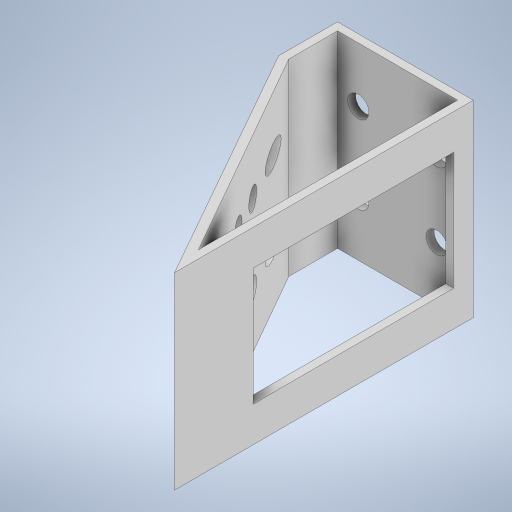
# Autodesk Inventor part: AngleMount
Saved by Autodesk Inventor 2024.2 (Build 282272000, 272)
## iProperties
Created: 2023-11-06
Part Number: AngleMount
Material: Generic
Document SubType Name: Modeling
Designer: S227943
Density: 1 g/cm^3
Appearance: Default
Author: S227943
Autodesk Inventor part; units mm, degrees
ref_plane "YZ Plane" through (0, 0, 0) normal (1, 0, 0) x (0, 1, 0)
ref_plane "XZ Plane" through (0, 0, 0) normal (0, 1, 0) x (-1, 0, 0)
ref_plane "XY Plane" through (0, 0, 0) normal (0, 0, 1) x (1, 0, 0)
sketch "Sketch1" plane through (0, 0, 0) normal (0, 1, 0) x (-1, 0, 0)
  line L0 (0, 0) -> (0, -19.05)
  line L1 (0, -19.05) -> (43.942, -19.05)
  line L2 (43.942, -19.05) -> (43.942, 0)
  line L3 (43.942, 0) -> (0, 0)
  line L4 (0, 0) -> (0, 155.3344)
  line L5 (43.942, 0) -> (0, 77.6672)
  dimension "d0" = 19.05
  dimension "d1" = 43.942
  dimension "d2" = 60.5
  constraints: 12 end point, 2 perpendicular, 2 vertical, 1 horizontal, 1 midpoint
  measures "d0" distance of L0.start L0.end
  measures "d1" distance of L0.end L1.end
  measures "d2" angle of L3 L5
extrude "Extrusion1" add sketch "Sketch1" along normal blind 60.96
sketch "Sketch6" plane through (0, 60.96, 0) normal (0, 1, 0) x (1, 0, 0)
  line L0 (0, 19.05) -> (-43.942, 19.05) projected
  line L1 (0, -76.952) -> (0, 19.05)
  line L2 (0, 19.05) -> (-43.942, 19.05)
  line L3 (-43.942, 19.05) -> (-43.942, 0.0548)
  line L4 (-43.942, 0.0548) -> (0, -76.952)
  line L5 (-2.54, -67.3758) -> (-2.54, 16.51)
  line L6 (-2.54, 16.51) -> (-41.402, 16.51)
  line L7 (-41.402, 16.51) -> (-41.402, 0.7285)
  line L8 (-41.402, 0.7285) -> (-2.54, -67.3758)
  point P0 (0, 0)
  dimension "d26" = 2.54
  constraints: 16 end point, 2 perpendicular, 1 collinear, 1 vertical, 3 other
  measures "d26" distance between parallel lines of L4 L8
extrude "Extrusion5" cut sketch "Sketch6" against normal blind 76.2 contours L8 L7 L6 L5
sketch "Sketch2" plane through (0, 0, 77.6672) normal (-0.8703557, 0, 0.4924236) x (0.4924236, 0, 0.8703557)
  line L0 (0, 60.96) -> (-84.1784, 60.96) projected
  line L1 (0, 60.96) -> (-14.1351, 60.96)
  line L2 (-14.1351, 60.96) -> (-14.1351, 0)
  line L3 (0, 0) -> (-84.1784, 0) projected
  line L4 (-14.1351, 60.96) -> (-75.0951, 60.96)
  line L5 (-75.0951, 60.96) -> (-75.0951, 0)
  line L6 (-75.0951, 0) -> (-14.1351, 0)
  line L7 (-14.1351, 60.96) -> (-44.6151, 60.96)
  line L8 (-44.6151, 60.96) -> (-44.6151, 0)
  line L9 (-75.0951, 30.48) -> (-14.1351, 30.48)
  line L10 (-44.6151, 30.48) -> (-19.6139, 30.48)
  line L11 (-44.6151, 30.48) -> (-31.9151, 30.48)
  line L12 (-31.9151, 30.48) -> (-31.9151, 43.18)
  line L13 (-31.9151, 43.18) -> (-44.6151, 43.18)
  line L14 (-44.6151, 43.18) -> (-57.3151, 43.18)
  line L15 (-57.3151, 43.18) -> (-57.3151, 30.48)
  line L16 (-57.3151, 30.48) -> (-57.3151, 17.78)
  line L17 (-57.3151, 17.78) -> (-44.6151, 17.78)
  line L18 (-44.6151, 17.78) -> (-31.9151, 17.78)
  line L19 (-31.9151, 30.48) -> (-31.9151, 17.78)
  circle A0 centre (-44.6151, 30.48) radius 3.429
  circle A1 centre (-31.9151, 30.48) radius 3.429
  circle A2 centre (-31.9151, 17.78) radius 3.429
  circle A3 centre (-44.6151, 17.78) radius 3.429
  circle A4 centre (-57.3151, 17.78) radius 3.429
  circle A5 centre (-57.3151, 30.48) radius 3.429
  circle A6 centre (-57.3151, 43.18) radius 3.429
  circle A7 centre (-44.6151, 43.18) radius 3.429
  circle A8 centre (-31.9151, 43.18) radius 3.429
  point P0 (-67.5981, 0)
  dimension "d5" = 14.1351
  dimension "d6" = 60.96
  dimension "d7" = 30.48
  dimension "d8" = 25.0012
  dimension "d9" = 12.7
  dimension "d10" = 12.7
  dimension "d11" = 12.7
  dimension "d12" = 12.7
  dimension "d29" = 6.858
  dimension "d30" = 6.858
  dimension "d31" = 6.858
  dimension "d32" = 6.858
  dimension "d33" = 6.858
  dimension "d34" = 6.858
  dimension "d35" = 6.858
  dimension "d36" = 6.858
  dimension "d37" = 6.858
  constraints: 36 end point, 12 point on line, 9 centre point, 9 coincident, 7 perpendicular, 5 midpoint
  measures "d5" distance of L0.start L1.end
  measures "d6" distance of L1.end L4.end
  measures "d7" distance of L1.end L7.end
  measures "d8" distance of L10.start L10.end
  measures "d9" distance of L10.start L11.end
  measures "d10" distance of L11.end L12.end
  measures "d11" distance of L13.end L14.end
  measures "d12" distance of L15.end L16.end
  measures "d29" diameter of A0
  measures "d30" diameter of A1
  measures "d31" diameter of A2
  measures "d32" diameter of A3
  measures "d33" diameter of A4
  measures "d34" diameter of A5
  measures "d35" diameter of A6
  measures "d36" diameter of A7
  measures "d37" diameter of A8
hole "Hole1" [suppressed]
extrude "Extrusion6" [suppressed]
sketch "Sketch7" plane through (0, 0, 77.6672) normal (1, 0, 0) x (0, 0, -1)
  line L0 (96.7172, 0) -> (96.7172, 60.96) projected
  line L1 (96.7172, 60.96) -> (96.7172, 0)
  line L2 (96.7172, 0) -> (19.1044, 0)
  line L3 (19.1044, 0) -> (19.1044, 60.96)
  line L4 (19.1044, 60.96) -> (96.7172, 60.96)
  line L5 (90.3672, 54.61) -> (90.3672, 6.35)
  line L6 (90.3672, 6.35) -> (25.4544, 6.35)
  line L7 (25.4544, 6.35) -> (25.4544, 54.61)
  line L8 (25.4544, 54.61) -> (90.3672, 54.61)
  point P0 (77.6672, 0)
  dimension "d40" = 6.35
  constraints: 16 end point, 6 perpendicular, 1 collinear, 3 other
  measures "d40" distance between parallel lines of L4 L8
extrude "Extrusion7" cut sketch "Sketch7" against normal blind 5.08 contours L5 L6 L7 L8
sketch "Sketch8" plane through (0, 0, -19.05) normal (0, 0, -1) x (-1, 0, 0)
  line L0 (41.402, 60.96) -> (2.54, 60.96) projected
  line L1 (21.971, 60.96) -> (21.971, 0)
  line L2 (21.971, 0) -> (21.9695, 30.48)
  line L3 (21.971, 0) -> (21.9695, 30.48)
  line L4 (21.9695, 30.48) -> (0, 30.48)
  line L5 (0, 30.48) -> (43.942, 30.48)
  line L6 (43.942, 0) -> (43.942, 60.96) projected
  line L7 (21.9695, 30.48) -> (34.6695, 30.48)
  line L8 (34.6695, 30.48) -> (34.6695, 43.18)
  line L9 (34.6695, 43.18) -> (9.2695, 43.18)
  line L10 (9.2695, 43.18) -> (9.2695, 17.78)
  line L11 (9.2695, 17.78) -> (34.6695, 17.78)
  circle A0 centre (9.2695, 42.4173) radius 3.429
  circle A1 centre (34.6695, 43.18) radius 3.429
  circle A2 centre (9.2695, 17.78) radius 3.429
  circle A3 centre (34.6695, 17.78) radius 3.429
  point P0 (0, 0)
  dimension "d43" = 12.7
  dimension "d44" = 12.7
  dimension "d45" = 25.4
  dimension "d47" = 25.4
  dimension "d48" = 25.4
  dimension "d49" = 6.858
  dimension "d50" = 6.858
  dimension "d51" = 6.858
  dimension "d52" = 6.858
  constraints: 20 end point, 4 centre point, 3 coincident, 3 perpendicular, 2 midpoint, 2 point on line, 2 vertical, 1 horizontal
  measures "d43" distance of L4.start L7.end
  measures "d44" distance of L7.end L8.end
  measures "d45" distance of L8.end L9.end
  measures "d47" distance of L9.end L10.end
  measures "d48" distance of L10.end L11.end
  measures "d49" diameter of A0
  measures "d50" diameter of A1
  measures "d51" diameter of A2
  measures "d52" diameter of A3
extrude "Extrusion8" [suppressed]
extrude "Extrusion9" cut sketch "Sketch8" against normal blind 101.6 contours A1 L8 L9 | L9 L8 A1 | A0 L10 L9 | L9 L10 A0 | A2 L10 L11 | L11 L10 A2 | A3
extrude "Extrusion10" cut sketch "Sketch2" against normal blind 25.4 contours A7 L13 L8 | L8 L14 A7 | L13 A7 L8 | L8 A7 L14 | A1 L19 L9 | L9 L12 A1 | A5 L15 L9 | L9 L16 A5 | A8 L12 L13 | L13 L12 A8 | A6 L15 L14 | L14 L15 A6 | A3 L17 L8 | L8 L18 A3 | L19 A1 L9 | L9 A1 L12 | L15 A5 L9 | L9 A5 L16 | A0 L9 L8 | L8 L9 A0 | L17 A3 L8 | L8 A3 L18 | A2 L18 L19 | L19 L18 A2 | A4 L17 L16 | L16 L17 A4 | L9 A0 L8 | L8 A0 L9
thicken "Thicken2" operation add thickness 5.08 both sides no extend neighbours no toward (0, -1, 0) faces at (-1.6933, 54.61, 30.5752)
thicken "Thicken3" operation add thickness 5.08 both sides no extend neighbours no toward (0, 1, 0) faces at (-0.8467, 6.35, 30.5752)
body "Solid1"
